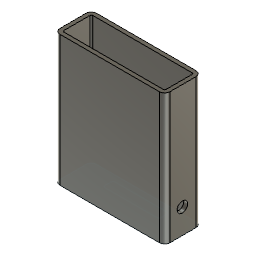
laptopStandV1 (Autodesk Fusion 360 design; units mm, degrees)
part number: 2026-02-23-19-42-26-801
Autodesk Fusion 360 part; units mm, degrees
sketch "Sketch1" plane through (0, 0, 0) normal (0, 0, 1) x (1, 0, 0)
  line L0 (22.7481, 79.1534) -> (232.7481, 79.1534)
  line L1 (232.7481, 79.1534) -> (232.7481, 9.1534)
  line L2 (232.7481, 9.1534) -> (22.7481, 9.1534)
  line L3 (22.7481, 9.1534) -> (22.7481, 79.1534)
  constraint horizontal L0
  constraint vertical L1
  constraint horizontal L2
  constraint vertical L3
extrude "Extrude1" add sketch "Sketch1" along normal blind 250
fillet "Fillet1" radius 10 1 edges at (22.7481, 9.1534, 125)
fillet "Fillet2" radius 10 1 edges at (232.7481, 9.1534, 125)
fillet "Fillet3" radius 10 1 edges at (22.7481, 79.1534, 125)
fillet "Fillet4" radius 10 1 edges at (232.7481, 79.1534, 125)
shell "Shell1" thickness 7.5 removed faces 1 at (159.4147, 32.4867, 250)
sketch "Sketch2" plane through (0, 0, 0) normal (0, 0, 1) x (1, 0, 0)
  line L0 (180.4304, 50.4408) -> (77.6973, 50.4408)
  line L1 (77.6973, 50.4408) -> (77.6973, 65.4408)
  line L2 (77.6973, 65.4408) -> (180.4304, 65.4408)
  line L3 (180.4304, 65.4408) -> (180.4304, 50.4408)
  line L4 (180.4304, 50.4408) -> (77.6973, 65.4408) construction
  line L5 (77.6973, 50.4408) -> (180.4304, 65.4408) construction
  point P0 (129.0638, 57.9408)
  constraint horizontal L0
  constraint perpendicular L0 L1
  constraint parallel L0 L2
  constraint parallel L1 L3
  constraint coincident L4 P0
  constraint coincident L5 P0
extrude "Extrude2" cut sketch "Sketch2" along normal blind 24
fillet "Fillet5" radius 2 12 edges at (129.0638, 65.4408, 0) (129.0638, 50.4408, 0) (77.6973, 57.9408, 0) (180.4304, 57.9408, 0) (77.6973, 50.4408, 3.75) (129.0638, 65.4408, 7.5) (77.6973, 57.9408, 7.5) (77.6973, 65.4408, 3.75) (180.4304, 50.4408, 3.75) (180.4304, 65.4408, 3.75) (180.4304, 57.9408, 7.5) (129.0638, 50.4408, 7.5) 4 faces at (77.6973, 55.4408, 2.5) (146.186, 50.4408, 2.5) (180.4304, 60.4408, 5) (111.9416, 65.4408, 2.5)
sketch "Sketch3" plane through (0, 0, 0) normal (0, 0, -1) x (1, 0, 0)
  arc A0 (222.7481, -79.1534) -> (232.7481, -69.1534) centre (222.7481, -69.1534) ccw
  line L0 (232.7481, -69.1534) -> (232.7481, -19.1534)
  arc A1 (232.7481, -19.1534) -> (222.7481, -9.1534) centre (222.7481, -19.1534) ccw
  line L1 (222.7481, -9.1534) -> (32.7481, -9.1534)
  arc A2 (32.7481, -9.1534) -> (22.7481, -19.1534) centre (32.7481, -19.1534) ccw
  line L2 (22.7481, -19.1534) -> (22.7481, -69.1534)
  arc A3 (22.7481, -69.1534) -> (32.7481, -79.1534) centre (32.7481, -69.1534) ccw
  line L3 (32.7481, -79.1534) -> (222.7481, -79.1534)
  arc A4 (178.4304, -67.4408) -> (182.4304, -63.4408) centre (178.4304, -63.4408) ccw
  line L4 (178.4304, -67.4408) -> (79.6973, -67.4408)
  arc A5 (75.6973, -63.4408) -> (79.6973, -67.4408) centre (79.6973, -63.4408) ccw
  line L5 (75.6973, -63.4408) -> (75.6973, -52.4408)
  arc A6 (79.6973, -48.4408) -> (75.6973, -52.4408) centre (79.6973, -52.4408) ccw
  line L6 (79.6973, -48.4408) -> (178.4304, -48.4408)
  arc A7 (182.4304, -52.4408) -> (178.4304, -48.4408) centre (178.4304, -52.4408) ccw
  line L7 (182.4304, -52.4408) -> (182.4304, -63.4408)
hole "Hole1" at (22.7481, 43.0604, 47.3957) direction (1, 0, 0) diameter 20 depth 300 tip angle 118
ref_plane "WorkPlane1" through (127.7481, 79.1534, 125) normal (0, 1, 0) x (-1, 0, 0)
sketch "Sketch4" plane through (0, 79.1534, 0) normal (0, 1, 0) x (1, 0, 0)
  line L0 (207.7481, -10) -> (185.6481, -10)
  line L1 (185.6481, -10) -> (185.6481, -237)
  line L2 (185.6481, -237) -> (207.7481, -237)
  line L3 (207.7481, -237) -> (207.7481, -10)
  line L4 (32.7481, 0) -> (222.7481, 0)
  line L5 (222.7481, 0) -> (222.7481, -250)
  line L6 (207.7481, -10) -> (185.6481, -10)
  line L7 (185.6481, -10) -> (185.6481, -237)
  line L8 (185.6481, -237) -> (207.7481, -237)
  line L9 (207.7481, -237) -> (207.7481, -10)
  line L10 (69.8481, -10) -> (47.7481, -10)
  line L11 (47.7481, -10) -> (47.7481, -237)
  line L12 (47.7481, -237) -> (69.8481, -237)
  line L13 (69.8481, -237) -> (69.8481, -10)
  line L14 (32.7481, -250) -> (32.7481, 0)
  dimension "d25" = 10
  dimension "d26" = 15
  dimension "d27" = 22.1
  dimension "d28" = 227
  dimension "d29" = 227
  dimension "d30" = 22.1
  dimension "d31" = 10
  dimension "d32" = 15
  constraint horizontal L0
  constraint vertical L1
  constraint horizontal L2
  constraint vertical L3
  constraint horizontal L6
  constraint vertical L7
  constraint horizontal L8
  constraint vertical L9
  constraint horizontal L10
  constraint vertical L11
  constraint horizontal L12
  constraint vertical L13
  measures "d25" distance of L0.end L4
  measures "d26" distance of L2.end L5
  measures "d27" distance of L2.end L1.end
  measures "d28" distance of L0.end L1.end
  measures "d29" distance of L10.end L11.end
  measures "d30" distance of L10.start L10.end
  measures "d31" distance of L4 L10.end
  measures "d32" distance of L11.end L14
extrude "Extrude3" cut sketch "Sketch4" against normal blind 3
